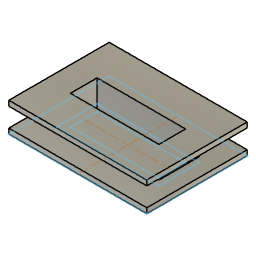
EE Core Bobbin Maker (Parameterized) (Autodesk Fusion 360 design; units mm, degrees)
part number: 2025-10-28-19-20-34-894
Autodesk Fusion 360 part; units mm, degrees
sketch "Sketch1" plane through (0, 0, 0) normal (0, 0, 1) x (1, 0, 0)
  line L0 (0.4589, 72.3441) -> (40.8589, 72.3441)
  line L1 (40.8589, 72.3441) -> (40.8589, 42.9441)
  line L2 (40.8589, 42.9441) -> (0.4589, 42.9441)
  line L3 (0.4589, 42.9441) -> (0.4589, 72.3441)
  line L4 (7.7089, 61.5441) -> (33.6089, 61.5441)
  line L5 (33.6089, 61.5441) -> (33.6089, 53.7441)
  line L6 (33.6089, 53.7441) -> (7.7089, 53.7441)
  line L7 (7.7089, 53.7441) -> (7.7089, 61.5441)
  line L8 (20.6589, 72.3441) -> (20.6589, 42.9441) construction
  line L9 (7.7089, 57.6441) -> (33.6089, 57.6441) construction
  line L10 (35.6089, 51.7441) -> (5.7089, 51.7441)
  line L11 (5.7089, 51.7441) -> (5.7089, 63.5441)
  line L12 (5.7089, 63.5441) -> (35.6089, 63.5441)
  line L13 (35.6089, 63.5441) -> (35.6089, 51.7441)
  dimension "d7" = 10.8
  dimension "d8" = 10.8
  dimension "d9" = 7.8
  dimension "d10" = 25.9
  dimension "d11" = 40.4
  dimension "d12" = -2
  constraint horizontal L0
  constraint vertical L1
  constraint horizontal L2
  constraint vertical L3
  constraint horizontal L4
  constraint vertical L5
  constraint horizontal L6
  constraint vertical L7
  constraint midpoint L0 L8.start
  constraint midpoint L2 L8.end
  constraint midpoint L7 L9.start
  constraint midpoint L5 L9.end
  constraint midpoint L8 L9
  measures "d7" distance of L0 L4
  measures "d8" distance of L2 L6
  measures "d9" distance of L4 L6
  measures "d10" distance of L5 L7
  measures "d11" distance of L1 L3
extrude "Extrude1" add sketch "Sketch1" along normal blind 8.55 contours L10 L11 L12 L13
extrude "Extrude2" add sketch "Sketch1" along normal blind 1.5 contours L0 L1 L2 L3
sketch "Sketch2" plane through (0, 0, 8.55) normal (0, 0, 1) x (-1, 0, 0)
  line L0 (-33.6089, -53.7441) -> (-7.7089, -53.7441)
  line L1 (-7.7089, -53.7441) -> (-7.7089, -61.5441)
  line L2 (-7.7089, -61.5441) -> (-33.6089, -61.5441)
  line L3 (-33.6089, -61.5441) -> (-33.6089, -53.7441)
  line L4 (-35.6089, -63.5441) -> (-5.7089, -63.5441)
  line L5 (-5.7089, -63.5441) -> (-5.7089, -51.7441)
  line L6 (-5.7089, -51.7441) -> (-35.6089, -51.7441)
  line L7 (-35.6089, -51.7441) -> (-35.6089, -63.5441)
  line L8 (-40.8589, -72.3441) -> (-40.8589, -42.9441)
  line L9 (-0.4589, -72.3441) -> (-40.8589, -72.3441)
  line L10 (-40.8589, -42.9441) -> (-0.4589, -42.9441)
  line L11 (-0.4589, -42.9441) -> (-0.4589, -72.3441)
extrude "Extrude3" add sketch "Sketch2" against normal blind 1.5 contours L8 L9 L10 L11
equation "CenterLegWidth = 7.3 mm"
equation "CenterLegThickness = 25.4 mm"
equation "SideLegWidth = 3.65 mm"
equation "SideLegThickness = 25.4 mm"
equation "WindowWidth = 11.6 mm"
equation "WindowHeight = 9 mm"
equation "d7 = WindowWidth - 0.8 mm"
equation "d8 = WindowWidth - 0.8 mm"
equation "d9 = CenterLegWidth + 0.5 mm"
equation "d10 = CenterLegThickness + 0.5 mm"
equation "d11 = CenterLegThickness + 15 mm"
equation "d13 = WindowHeight - 0.45 mm"
